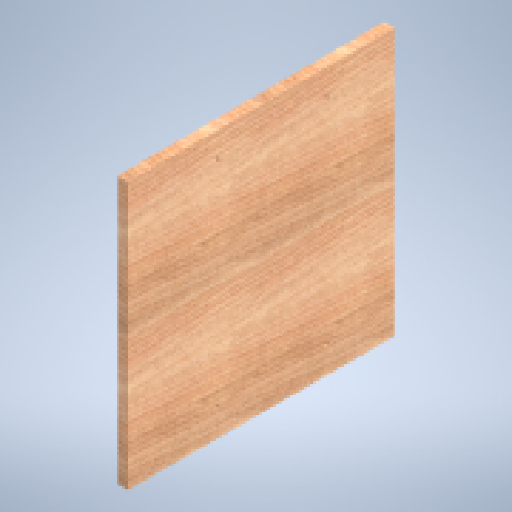
# Autodesk Inventor part: Sitzplatte
Saved by Autodesk Inventor 2024.4 (Build 284460000, 460)
## iProperties
Created: 2026-01-11
Part Number: Sitzplatte
Material: Holz (Birke)
Description: Sitzplatte
Document SubType Name: Modeling
Designer: julia
Mass: 2743.73 g
Surface Area: 5437.11 cm^2
Volume: 4988.6 cm^3
Density: 0.55 g/cm^3
Appearance: Birke - natur - poliert
DocNumber: Sitzplatte.ipt
Folder: I60-Konstruktion\I60-Gruppe-7\Sitz\
VDS_Category: Konstruktion
Masse[kg]: 2,745 kg
Autodesk Inventor part; units mm, degrees
ref_plane "YZ Plane" through (0, 0, 0) normal (1, 0, 0) x (0, 1, 0)
ref_plane "XZ Plane" through (0, 0, 0) normal (0, 1, 0) x (-1, 0, 0)
ref_plane "XY Plane" through (0, 0, 0) normal (0, 0, 1) x (1, 0, 0)
sketch "Skizze1" plane through (0, 0, 0) normal (1, 0, 0) x (0, 1, 0)
  line L0 (-250, 250) -> (250, 250)
  line L1 (250, 250) -> (250, -250)
  line L2 (250, -250) -> (-250, -250)
  line L3 (-250, -250) -> (-250, 250)
  line L4 (-250, 250) -> (250, -250) construction
  line L5 (250, 250) -> (-250, -250) construction
  point P0 (0, 0)
  dimension "d0" = 500
  dimension "d1" = 500
  constraints: 12 end point, 2 midpoint, 2 parallel, 1 horizontal, 1 perpendicular
  measures "d0" distance of L1.end L2.end
  measures "d1" distance of L0.end L1.end
extrude "Extrusion1" add sketch "Skizze1" along normal blind 20
sketch "Skizze2" plane through (0, 0, 0) normal (-1, 0, 0) x (0, 0, 1)
  line L0 (0, 0) -> (0, -82)
  line L1 (0, -82) -> (200, -82)
  line L2 (200, -82) -> (-200, -82)
  line L3 (-200, -82) -> (-200, 122)
  line L4 (-200, 122) -> (200, 122)
  dimension "d4" = 82
  dimension "d5" = 200
  dimension "d71" = 204
  dimension "d72" = 400
  constraints: 10 end point, 1 horizontal, 1 perpendicular, 1 point on line, 1 vertical, 1 vertical alignment, 4 other
  measures "d4" distance of L0.start L0.end
  measures "d5" distance of L0.end L1.end
  measures "d71" distance of L2.end L3.end
  measures "d72" distance of L3.end L4.end
hole "Bohrung1" at (0, -82, 200) at (0, -82, -200) at (0, 122, 200) at (0, 122, -200) direction (1, 0, 0) diameter 10.5 end through all countersink diameter 21 countersink angle 90
sketch "Skizze4" plane through (0, 250, 250) normal (0, 1, 0) x (1, 0, 0)
  line L0 (0, 0) -> (20, 0) projected
  line L1 (0, 0) -> (0, 85)
  line L2 (0, 500) -> (0, 0) projected
  line L3 (20, 0) -> (8, 0)
  line L4 (8, 0) -> (8, 85)
  line L5 (8, 85) -> (8, 97)
  line L6 (8, 97) -> (8, 133)
  line L7 (20, 500) -> (20, 0) projected
  line L8 (20, 500) -> (8, 500)
  line L9 (0, 500) -> (20, 500) projected
  line L10 (8, 500) -> (8, 415)
  line L11 (8, 415) -> (8, 403)
  line L12 (8, 403) -> (8, 367)
  point P0 (0, 250)
  dimension "d40" = 12
  dimension "d41" = 85
  dimension "d42" = 12
  dimension "d43" = 36
  dimension "d44" = 12
  dimension "d45" = 85
  dimension "d46" = 12
  dimension "d47" = 36
  constraints: 18 end point, 7 point on line, 1 perpendicular, 1 vertical
  measures "d40" distance of L0.end L3.end
  measures "d41" distance of L3.end L4.end
  measures "d42" distance of L4.end L5.end
  measures "d43" distance of L5.end L6.end
  measures "d44" distance of L7.start L8.end
  measures "d45" distance of L8.end L10.end
  measures "d46" distance of L10.end L11.end
  measures "d47" distance of L11.end L12.end
hole "Bohrung2" at (8, 250, 153) at (8, 250, 117) at (8, 250, -117) at (8, 250, -153) direction (0, -1, 0) diameter 4 depth 20 tip angle 118
sketch "Skizze5" plane through (0, 250, 250) normal (0, 1, 0) x (1, 0, 0)
  line L0 (0, 0) -> (0, 500) projected
  line L1 (0, 0) -> (10, 0)
  line L2 (0, 0) -> (20, 0) projected
  line L3 (10, 0) -> (10, 30)
  line L4 (10, 0) -> (10, 190)
  line L5 (0, 500) -> (10, 500)
  line L6 (0, 500) -> (20, 500) projected
  line L7 (10, 500) -> (-20, 500)
  line L8 (10, 500) -> (10, 470)
  line L9 (10, 500) -> (10, 310)
  point P0 (0, 250)
  dimension "d55" = 10
  dimension "d56" = 30
  dimension "d57" = 190
  dimension "d58" = 10
  dimension "d59" = 30
  dimension "d60" = 30
  dimension "d61" = 190
  constraints: 14 end point, 3 vertical, 2 midpoint, 1 perpendicular, 1 point on line
  measures "d55" distance of L0.start L1.end
  measures "d56" distance of L1.end L3.end
  measures "d57" distance of L1.end L4.end
  measures "d58" distance of L0.end L5.end
  measures "d59" distance of L5.end L7.end
  measures "d60" distance of L5.end L8.end
  measures "d61" distance of L5.end L9.end
hole "Bohrung3" at (10, 250, 220) at (10, 250, 60) at (10, 250, -60) at (10, 250, -220) direction (0, -1, 0) diameter 4 depth 20 tip angle 118
